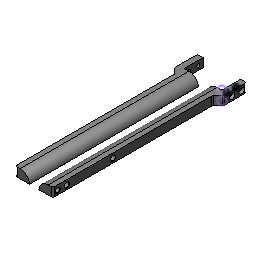
Ramp_Extension (Autodesk Fusion 360 design; units mm, degrees)
Autodesk Fusion 360 part; units mm, degrees
sketch "Sketch1" plane through (0, 0, 0) normal (0, 0, 1) x (1, 0, 0)
  line L0 (5, 0) -> (20, 0)
  line L1 (20, 0) -> (20, -180)
  line L2 (20, -180) -> (5, -180)
  line L3 (5, -180) -> (5, 0)
  line L4 (20, -10) -> (26, -4)
  line L5 (20, -10) -> (30.8245, -10) construction
  line L6 (26, -4) -> (26, 20)
  line L7 (26, 20) -> (20, 20)
  line L8 (20, 20) -> (20, 0)
  line L9 (0, 0) -> (5, 0) construction
  dimension "d1" = 15
  dimension "d2" = 180
  dimension "d3" = 45
  dimension "d4" = 10
  dimension "d5" = 200
  dimension "d6" = 6
  dimension "d31" = 5
  constraint horizontal L0
  constraint vertical L1
  constraint horizontal L2
  constraint vertical L3
  constraint horizontal L5
  constraint coincident L1 L4.start
  constraint vertical L6
  constraint perpendicular L6 L7
  constraint perpendicular L0 L8
  constraint coincident L9.start origin
  constraint perpendicular L8 L9
  constraint coincident L0.start L3.end
  measures "d1" distance of L0.start L0.end
  measures "d2" distance of L0.start L2.end
  measures "d3" angle of L4 L5
  measures "d4" distance of L0 L4.start
  measures "d5" distance of L2 L7
  measures "d6" distance of L6 L8
  measures "d31" distance of L9.start L0.start
extrude "Extrude1" add sketch "Sketch1" along normal blind 10 makes body 1
sketch "Sketch2" plane through (20, 0, 0) normal (-1, 0, 0) x (0, -1, 0)
  line L0 (-20, 0) -> (0, 0)
  line L1 (0, 0) -> (0, 10)
  line L2 (0, 10) -> (-20, 10)
  line L3 (-20, 10) -> (-20, 0)
  circle A0 centre (-15, 5) radius 1.75
  circle A1 centre (-15, 5) radius 3
  line L4 (-20, 5) -> (0, 5) construction
  line L5 (-10, 5) -> (-10, 10) construction
  circle A2 centre (-5, 5) radius 1.75
  circle A3 centre (-5, 5) radius 3
  line L6 (0, 0) -> (0, 10) construction
  dimension "d9" = 3.5
  dimension "d10" = 6
  dimension "d11" = 5
  constraint concentric A0 A1
  constraint midpoint L3 L4.start
  constraint midpoint L1 L4.end
  constraint midpoint L4 L5.start
  constraint midpoint L2 L5.end
  constraint symmetric A0 L5 A2
  constraint symmetric A1 L5 A3
  constraint coincident A0.centre L4
  measures "d9" diameter of A0
  measures "d10" diameter of A1
  measures "d11" distance of A2.centre L6
extrude "Extrude2" cut sketch "Sketch2" against normal up to surface (6 mm away) contours A0 | A2 bodies 1
extrude "Extrude3" cut sketch "Sketch2" along normal blind 3 from surface at -6 contours A1 | A3 bodies 1
sketch "Sketch3" plane through (20, 0, 0) normal (1, 0, 0) x (0, 1, 0)
  line L0 (-180, 0) -> (-10, 0)
  line L1 (-10, 0) -> (-10, 10)
  line L2 (-10, 10) -> (-180, 10)
  line L3 (-180, 10) -> (-180, 0)
  line L4 (-180, 5) -> (-93.8269, 5) construction
  circle A0 centre (-175, 5) radius 2.35
  circle A1 centre (-165, 5) radius 2.35
  circle A2 centre (-115.665, 5) radius 2.35
  dimension "d17" = 4.7
  dimension "d18" = 4.7
  dimension "d19" = 10
  dimension "d20" = 5
  dimension "d23" = 4.7
  dimension "d24" = 64.335
  constraint midpoint L3 L4.start
  constraint perpendicular L3 L4
  constraint coincident L4 A0.centre
  constraint coincident L4 A1.centre
  constraint coincident L4 A2.centre
  measures "d17" diameter of A0
  measures "d18" diameter of A1
  measures "d19" distance of A0.centre A1.centre
  measures "d20" distance of L3 A0.centre
  measures "d23" diameter of A2
  measures "d24" distance of L3 A2.centre
extrude "Extrude4" cut sketch "Sketch3" against normal blind 6 contours A0 | A1 | A2 bodies 1
fillet "Fillet1" radius 10 1 edges at (5, -90, 10) on bodies 1
fillet "Fillet2" radius 2 3 edges at (20, -10, 5) (26, -4, 5) (26, 20, 5) on bodies 1
chamfer "Chamfer1" distance 0.4 angle 45 3 edges at (20, -177.191, 5.8498) (20, -167.191, 5.8498) (20, -117.856, 5.8498) on bodies 1
fillet "Fillet3" radius 2 1 edges at (20, -180, 5) on bodies 1
chamfer "Chamfer2" distance 0.6 angle 45 1 faces at (10, -63.6095, 0) on bodies 1
mirror "Mirror1" about plane through (0, 0, 0) normal (1, 0, 0) of bodies 1 makes body 2
